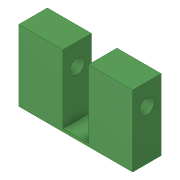
# Autodesk Inventor part: Kermit MountConnectors
Saved by Autodesk Inventor 2018.2 (Build 222227000, 227)
## iProperties
Created: 2018-03-05
Part Number: Kermit MountConnectors
Material: Generic
Document SubType Name: Modeling
Designer: lopez.xavier
Density: 1 g/cm^3
Appearance: Smooth - Dark Forest Green
Author: lopez.xavier
Autodesk Inventor part; units mm, degrees
ref_plane "YZ Plane" through (0, 0, 0) normal (1, 0, 0) x (0, 1, 0)
ref_plane "XZ Plane" through (0, 0, 0) normal (0, 1, 0) x (-1, 0, 0)
ref_plane "XY Plane" through (0, 0, 0) normal (0, 0, 1) x (1, 0, 0)
sketch "Sketch1" plane through (0, 0, 0) normal (0, 0, 1) x (1, 0, 0)
  line L0 (0, 0) -> (101.6, 0)
  line L1 (101.6, 0) -> (101.6, 63.5)
  line L2 (101.6, 63.5) -> (0, 63.5)
  line L3 (0, 63.5) -> (0, 0)
  dimension "d0" = 101.6
  dimension "d1" = 63.5
  constraints: 8 end point, 2 parallel, 1 horizontal, 1 perpendicular
  measures "d0" distance of L2.end L1.end
  measures "d1" distance of L1.end L0.end
extrude "Extrusion1" add sketch "Sketch1" along normal blind 25.4
sketch "Sketch2" plane through (101.6, 0, 0) normal (1, 0, 0) x (0, 0, -1)
  circle A0 centre (-12.7, 44.45) radius 6.35
  line L0 (-25.4, 0) -> (-25.4, 63.5) projected
  line L1 (0, 0) -> (-25.4, 0) projected
  line L2 (0, 63.5) -> (-25.4, 63.5) projected
  dimension "d4" = 12.7
  dimension "d5" = 12.7
  dimension "d13" = 19.05
  constraints: 1 centre point
  measures "d4" diameter of A0
  measures "d5" distance from line of L0 A0.centre
  measures "d13" distance from line of L2 A0.centre
extrude "Extrusion2" cut sketch "Sketch2" against normal blind 101.6
sketch "Sketch3" plane through (0, 63.5, 0) normal (0, 1, 0) x (1, 0, 0)
  line L0 (0, -25.4) -> (101.6, -25.4) projected
  line L1 (0, 0) -> (101.6, 0) projected
  line L2 (39.37, -25.4) -> (62.23, -25.4)
  line L3 (62.23, -25.4) -> (62.23, 0)
  line L4 (62.23, 0) -> (39.37, 0)
  line L5 (39.37, 0) -> (39.37, -25.4)
  line L6 (101.6, 0) -> (101.6, -25.4) projected
  dimension "d9" = 22.86
  dimension "d10" = 39.37
  constraints: 8 end point, 2 parallel, 2 point on line, 1 horizontal, 1 perpendicular
  measures "d9" distance of L4.end L3.end
  measures "d10" distance between parallel lines of L6 L3
extrude "Extrusion3" cut sketch "Sketch3" against normal blind 60.96 contours L5 L1 L3 L0
body "Solid1"
